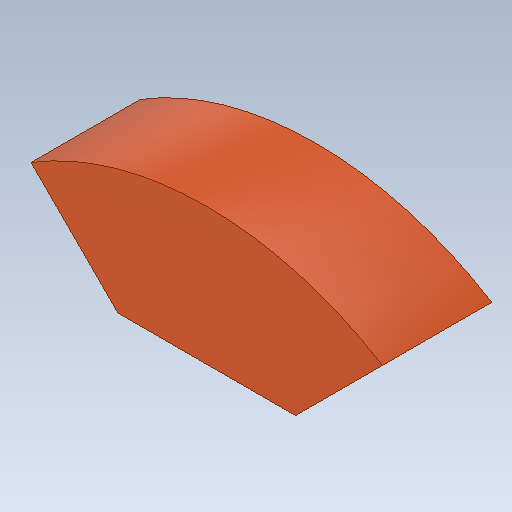
# Autodesk Inventor part: Calliper
Saved by Autodesk Inventor 2020 (Build 240168000, 168)
## iProperties
Created: 2020-09-30
Part Number: Calliper
Material: Steel, Alloy
Document SubType Name: Modeling
Designer: Federico
Density: 7.73 g/cm^3
Appearance: Smooth - Light Orange
Author: Federico
Autodesk Inventor part; units mm, degrees
sketch "Sketch1" plane through (0, 0, 0) normal (0, 0, 1) x (1, 0, 0)
  line L0 (0, 0) -> (130, 0)
  line L1 (130, 0) -> (193.6396, 63.6396)
  line L2 (0, 0) -> (-63.6396, 63.6396)
  arc A0 (193.6396, 63.6396) -> (-63.6396, 63.6396) centre (65, -144.7193) ccw
  dimension "d0" = 130
  dimension "d1" = 90
  dimension "d2" = 135
  dimension "d3" = 90
  constraints: 6 end point, 2 point on circle, 1 centre point, 1 horizontal
  measures "d0" distance of L0.start L0.end
  measures "d1" distance of L0.end L1.end
  measures "d2" angle of L1 L0
  measures "d3" distance of L0.start L2.end
extrude "Extrusion1" add sketch "Sketch1" along normal blind 80
ref_plane "Work Plane1" through (0, 0, 80) normal (0, 0, 1) x (1, 0, 0)
sketch "Sketch2" plane through (0, 0, 80) normal (0, 0, 1) x (1, 0, 0)
  line L0 (-63.6396, 63.6396) -> (0, 0) projected
  line L1 (0, 0) -> (-42.4264, 42.4264)
  line L2 (0, 0) -> (130, 0) projected
  line L3 (0, 0) -> (130, 0)
  line L4 (130, 0) -> (172.4264, 42.4264)
  line L5 (130, 0) -> (193.6396, 63.6396) projected
  arc A0 (172.4264, 42.4264) -> (-42.4264, 42.4264) centre (65, -155.2225) ccw
  dimension "d7" = 60
  dimension "d8" = 60
  constraints: 6 end point, 2 point on circle, 2 point on line, 1 centre point, 1 horizontal
  measures "d7" distance of L0.end L1.end
  measures "d8" distance of L2.end L4.end
extrude "Extrusion2" cut sketch "Sketch2" against normal blind 30
ref_plane "Work Plane2" through (0, 0, 0) normal (0, -1, 0) x (1, 0, 0)
sketch "Sketch4" plane through (0, 0, 0) normal (0, -1, 0) x (1, 0, 0)
  line L0 (-42.4264, 50) -> (-42.4264, 80) projected
  line L1 (-42.4264, 70) -> (172.4264, 70)
  line L2 (172.4264, 80) -> (172.4264, 50) projected
  line L3 (172.4264, 70) -> (172.4264, 80)
  line L4 (172.4264, 80) -> (-42.4264, 80)
  line L5 (193.6396, 80) -> (-63.6396, 80) projected
  line L6 (130, 50) -> (0, 50) projected
  point P0 (0, 0)
  dimension "d12" = 20
  constraints: 6 end point, 2 point on line, 1 collinear, 1 perpendicular
  measures "d12" distance between parallel lines of L6 L1
extrude "Extrusion3" add sketch "Sketch4" against normal blind 70
ref_plane "Work Plane3" through (0, 0, 0) normal (0, 0, -1) x (-1, 0, 0)
sketch "Sketch5" plane through (0, 0, 0) normal (0, 0, -1) x (-1, 0, 0)
  line L0 (-172.4264, 0) -> (-172.4264, 42.4264) projected
  line L1 (-172.4264, 42.4264) -> (-130, 0) projected
  line L2 (-172.4264, 0) -> (-172.4264, 42.4264)
  line L3 (-172.4264, 42.4264) -> (-130, 0)
  line L4 (42.4264, 0) -> (-172.4264, 0) projected
  line L5 (-130, 0) -> (-172.4264, 0)
  line L6 (-130, 0) -> (0, 0) projected
  line L7 (42.4264, 42.4264) -> (42.4264, 0)
  line L8 (63.6396, 63.6396) -> (0, 0) projected
  line L9 (42.4264, 42.4264) -> (0, 0)
  line L10 (0, 0) -> (42.4264, 0)
  constraints: 12 end point, 4 collinear, 1 perpendicular, 1 vertical
extrude "Extrusion4" cut sketch "Sketch5" against normal blind 80
ref_plane "Work Plane4" through (-63.6396, 63.6396, 80) normal (-0.7071, -0.7071, 0) x (-0.7071, 0.7071, 0)
sketch "Sketch6" plane through (-63.6396, 63.6396, 80) normal (-0.7071, -0.7071, 0) x (-0.7071, 0.7071, 0)
  circle A0 centre (-20.8328, 61.1519) radius 17
  circle A1 centre (-67.5207, 61.1519) radius 17
  point P0 (-90, 80)
  dimension "d19" = 34
  dimension "d21" = 34
  constraints: 2 centre point
  measures "d19" diameter of A0
  measures "d21" diameter of A1
extrude "Extrusion5" add sketch "Sketch6" along normal blind 15
sketch "Sketch7" plane through (-59.5152, 38.302, 18.8481) normal (-0.7071, -0.7071, 0) x (-0.7071, 0.7071, 0)
  circle A0 centre (0, 0) radius 12.5
  circle A1 centre (-46.6879, 0) radius 17 projected
  circle A2 centre (-46.6879, 0) radius 12.5
  point P0 (-69.1672, 18.8481)
  dimension "d24" = 25
  dimension "d25" = 25
  constraints: 2 centre point, 1 coincident
  measures "d24" diameter of A0
  measures "d25" diameter of A2
extrude "Extrusion6" cut sketch "Sketch7" against normal blind 20 contours A0
sketch "Sketch8" plane through (-26.5019, 5.2887, 18.8481) normal (-0.7071, -0.7071, 0) x (-0.7071, 0.7071, 0)
  circle A0 centre (0, 0) radius 12.5
  point P0 (-22.4793, 18.8481)
  dimension "d28" = 25
  constraints: 1 centre point
  measures "d28" diameter of A0
extrude "Extrusion7" cut sketch "Sketch8" against normal blind 20
body "Solid1"
